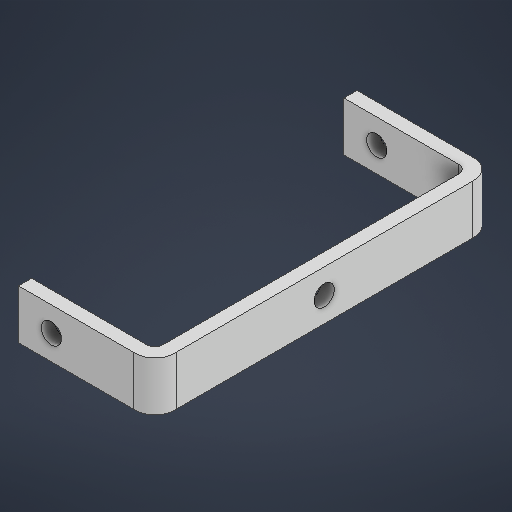
# Autodesk Inventor part: Side bar holding bracket
Saved by Autodesk Inventor 2027 (Build 310192000, 192)
## iProperties
Created: 2026-04-16
Part Number: Side bar holding bracket
Material: Generic
Document SubType Name: Modeling
Designer: ratik
Density: 1 g/cm^3
Appearance: Default
Author: ratik
Autodesk Inventor part; units mm, degrees
ref_plane "YZ Plane" through (0, 0, 0) normal (1, 0, 0) x (0, 1, 0)
ref_plane "XZ Plane" through (0, 0, 0) normal (0, 1, 0) x (-1, 0, 0)
ref_plane "XY Plane" through (0, 0, 0) normal (0, 0, 1) x (1, 0, 0)
sketch "Sketch1" plane through (0, 0, 0) normal (0, 1, 0) x (-1, 0, 0)
  line L0 (-16.7652, 6.8702) -> (-16.7652, -83.1298)
  line L1 (-12.7652, -83.1298) -> (-12.7652, 6.8702)
  line L2 (24.7348, -85.6298) -> (-10.2652, -85.6298)
  line L3 (-10.2652, -89.6298) -> (24.7348, -89.6298)
  line L4 (24.7348, -89.6298) -> (24.7348, -85.6298)
  line L5 (24.7348, 13.3702) -> (-10.2652, 13.3702)
  line L6 (-10.2652, 9.3702) -> (24.7348, 9.3702)
  line L7 (24.7348, 9.3702) -> (24.7348, 13.3702)
  arc A0 (-10.2652, 13.3702) -> (-16.7652, 6.8702) centre (-10.788, 7.3931) ccw
  arc A1 (-16.7652, -83.1298) -> (-10.2652, -89.6298) centre (-10.788, -83.6526) ccw
  arc A2 (-10.2652, 9.3702) -> (-12.7652, 6.8702) centre (-10.2652, 6.8702) ccw
  arc A3 (-12.7652, -83.1298) -> (-10.2652, -85.6298) centre (-10.2652, -83.1298) ccw
  point P0 (0, 0)
  dimension "d0" = 90
  dimension "d1" = 4
  dimension "d2" = 4
  dimension "d3" = 4
  dimension "d4" = 35
  dimension "d5" = 35
  dimension "d11" = 6
  dimension "d13" = 6
  dimension "d15" = 2.5
  dimension "d16" = 2.5
  constraints: 16 end point, 8 point on circle, 4 centre point, 3 parallel, 2 horizontal
  measures "d0" distance of L1.start L1.end
  measures "d1" distance of L1.end L0.start
  measures "d2" distance of L3.end L2.start
  measures "d3" distance of L6.end L5.start
  measures "d4" distance of L6.start L6.end
  measures "d5" distance of L3.start L3.end
  measures "d11" radius of A0
  measures "d13" radius of A1
  measures "d15" radius of A2
  measures "d16" radius of A3
extrude "Extrusion1" add sketch "Sketch1" along normal blind 15
sketch "Sketch2" plane through (-24.7348, 0, 13.3702) normal (0, 0, 1) x (1, 0, 0)
  circle A0 centre (10, 7.5) radius 3.1
  line L0 (0, 15) -> (35, 15) projected
  line L1 (0, 0) -> (0, 15) projected
  point P0 (24.7348, 0)
  dimension "d19" = 6.2
  dimension "d20" = 7.5
  dimension "d21" = 10
  constraints: 1 centre point
  measures "d19" diameter of A0
  measures "d20" distance from line of L0 A0.centre
  measures "d21" distance from line of L1 A0.centre
extrude "Extrusion2" cut sketch "Sketch2" against normal blind 120
sketch "Sketch3" plane through (12.7652, 0, -83.1298) normal (-1, 0, 0) x (0, 0, 1)
  circle A0 centre (45, 7.5) radius 3.1
  line L0 (0, 15) -> (90, 15) projected
  line L1 (-6.5, 0) -> (-6.5, 15) projected
  point P0 (83.1298, 0)
  dimension "d24" = 6.2
  dimension "d25" = 7.5
  dimension "d26" = 51.5
  constraints: 1 centre point
  measures "d24" diameter of A0
  measures "d25" distance from line of L0 A0.centre
  measures "d26" distance from line of L1 A0.centre
extrude "Extrusion3" cut sketch "Sketch3" against normal blind 120
body "Solid1"
